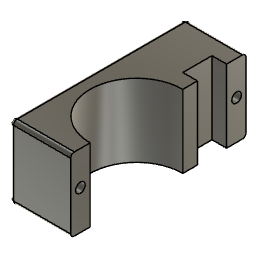
EmpurraBracoGK_12_Imprimir (Autodesk Fusion 360 design; units mm, degrees)
Autodesk Fusion 360 part; units mm, degrees
note: some values were not read from the file. Set by a fixed rule: which sketch regions a step uses.
sketch "Esboço1" plane through (0, 0, 0) normal (0, 0, 1) x (1, 0, 0)
  line L0 (15, 50.1) -> (21, 50.1)
  line L1 (15, 62.1) -> (15, 50.1)
  line L2 (-4, -2.1) -> (-4, 70.1)
  line L3 (-4, -2.1) -> (21, -2.1)
  line L4 (21, 70.1) -> (21, 62.1)
  line L5 (21, 62.1) -> (15, 62.1)
  line L6 (21, 5.9) -> (21, -2.1)
  line L7 (21, 50.1) -> (21, 44.1)
  arc A0 (21, 44.1) -> (21, 5.9) centre (21, 25) ccw
  line L8 (-4, 70.1) -> (21, 70.1)
  dimension "d2" = 12
  dimension "d3" = 6
  dimension "d5" = 8
  dimension "d8" = 6
  dimension "d10" = 8
  dimension "d36" = 25
  dimension "d12" = 6
  dimension "d13" = 19.1
  constraint perpendicular L4 L5
  constraint perpendicular L1 L5
  constraint perpendicular L0 L1
  constraint vertical L6
  constraint perpendicular L3 L6
  constraint perpendicular L0 L7
  measures "d2" distance of L1.start L0.start
  measures "d3" distance of L4.end L1.start
  measures "d5" distance of L4.end L4.start
  measures "d8" distance of L0.start L0.end
  measures "d10" distance of L6.start L3.end
  measures "d36" distance of L4.start L2.end
  measures "d12" distance of L0.end L7.end
  measures "d13" distance of L7.end A0.centre
extrude "Extrusão1" add sketch "Esboço1" along normal blind 30
hole "Furo1" at (-4, 66.2367, 16) direction (1, 0, 0) diameter 4 depth 25 tip angle 180
hole "Furo2" at (-4, 1.9, 16) direction (1, 0, 0) diameter 4 depth 25 tip angle 180
fillet "Arredondamento1" radius 1.5 5 edges at (-4, 34, 30) (-4, -2.1, 15) (8.5, -2.1, 30) (8.5, -2.1, 0) (-4, 34, 0)
fillet "Arredondamento2" radius 1.5 5 edges at (9.25, 70.1, 30) (-3.5607, 70.1, 29.5607) (-4, 70.1, 15) (-3.5607, 70.1, 0.4393) (9.25, 70.1, 0)
